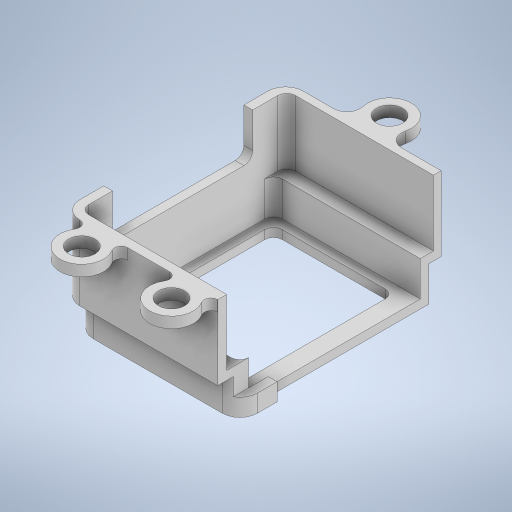
# Autodesk Inventor part: CO-1-06-motorControllersMount
Saved by Autodesk Inventor 2023 (Build 270158000, 158)
## iProperties
Created: 2023-01-24
Part Number: CO-1-06-motorControllersMount
Material: Generic
Document SubType Name: Modeling
Designer: t205b
Density: 1 g/cm^3
Appearance: Default
Author: t205b
Autodesk Inventor part; units mm, degrees
ref_plane "YZ Plane" through (0, 0, 0) normal (1, 0, 0) x (0, 1, 0)
ref_plane "XZ Plane" through (0, 0, 0) normal (0, 1, 0) x (-1, 0, 0)
sketch "Sketch1" plane through (0, 0, 0) normal (0, 1, 0) x (-1, 0, 0)
  arc A0 (31.569, 13.7227) -> (30.069, 12.2227) centre (31.569, 12.2227) ccw
  line L0 (31.569, 13.7227) -> (34.069, 13.7227)
  line L1 (34.069, 13.7227) -> (34.069, 18.9227)
  line L2 (32.069, 20.9227) -> (2.569, 20.9227)
  line L3 (34.069, -13.2773) -> (31.569, -13.2773)
  arc A1 (30.069, -11.7773) -> (31.569, -13.2773) centre (31.569, -11.7773) ccw
  arc A2 (34.069, 18.9227) -> (32.069, 20.9227) centre (32.069, 18.9227) ccw
  arc A3 (34.0195, 22.4149) -> (32.069, 23.9727) centre (32.069, 21.9727) ccw
  line L4 (32.069, 23.9727) -> (-23.931, 23.9727)
  arc A4 (-23.931, 23.9727) -> (-25.931, 21.9727) centre (-23.931, 21.9727) ccw
  line L5 (-25.931, 21.9727) -> (-25.931, -21.0273)
  arc A5 (-25.931, -21.0273) -> (-23.931, -23.0273) centre (-23.931, -21.0273) ccw
  line L6 (-23.931, -23.0273) -> (32.069, -23.0273)
  arc A6 (32.069, -23.0273) -> (33.899, -21.8341) centre (32.069, -21.0273) ccw
  arc A7 (32.069, -20.2773) -> (34.069, -18.2773) centre (32.069, -18.2773) ccw
  line L7 (32.069, -20.2773) -> (0.569, -20.2773)
  line L8 (34.069, -13.2773) -> (34.069, 13.7227)
  line L9 (0.569, -22.2773) -> (0.569, 18.9227)
  line L10 (30.069, -11.7773) -> (30.069, 12.2227)
  line L11 (34.069, -18.2773) -> (34.069, -13.2773)
  line L12 (2.569, 22.9227) -> (32.069, 22.9227)
  line L13 (0.569, -22.2773) -> (32.069, -22.2773)
  arc A8 (32.069, -22.2773) -> (36.069, -18.2773) centre (32.069, -18.2773) ccw
  line L14 (36.069, -18.2773) -> (36.069, 18.9227)
  arc A9 (2.569, 20.9227) -> (0.569, 18.9227) centre (2.569, 18.9227) ccw
  line L15 (-1.431, 14.4227) -> (-1.431, 18.9227)
  arc A10 (2.569, 22.9227) -> (-1.431, 18.9227) centre (2.569, 18.9227) ccw
  arc A11 (36.069, 18.9227) -> (32.069, 22.9227) centre (32.069, 18.9227) ccw
  line L16 (-1.431, 14.4227) -> (0.569, 14.4227)
  point P0 (0.569, 20.9227)
  dimension "d8" = 2
  dimension "d9" = 2
  dimension "d66" = 2
  dimension "d67" = 2
  dimension "d68" = 4.5
  dimension "d69" = 4
  constraints: 35 end point, 27 point on circle, 12 centre point, 8 vertical, 6 horizontal, 4 point on line, 3 tangent, 2 perpendicular, 1 collinear, 9 other
  measures "d8" distance between parallel lines of L2 L12
  measures "d9" distance between parallel lines of L7 L13
  measures "d66" radius of A9
  measures "d67" radial gap between concentric circles of A9 A10
  measures "d68" distance of L15.start L15.end
  measures "d69" radius of A11
extrude "Extrusion3" add sketch "Sketch1" against normal blind 2 contours L0 L8 L3 A1 L10 A0 | A0 L10 A1 L3 L11 A7 L7 L9 A9 L2 A2 L1 L0 | L1 A2 L2 A9 L9 L16 L15 A10 L12 A11 L14 A8 L13 L7 A7 L11 L8
ref_plane "Work Plane1" through (0, 8, 0) normal (0, 1, 0) x (1, 0, 0)
extrude "Extrusion4" add sketch "Sketch1" along normal blind 8 contours L1 A2 L2 A9 L9 L16 L15 A10 L12 A11 L14 A8 L13 L7 A7 L11 L8
sketch "Sketch2" plane through (0, 8, 0) normal (0, 1, 0) x (1, 0, 0)
  line L0 (-0.569, 22.2773) -> (-0.569, 22.2773) projected
  line L1 (-0.569, 22.2773) -> (-0.569, 22.2773)
  line L2 (-36.069, -21.9727) -> (-36.069, 21.0273)
  line L3 (-32.069, -25.9727) -> (-0.569, -25.9727)
  line L4 (-0.569, -14.4227) -> (-0.569, -18.9227) projected
  line L5 (-0.569, -25.9727) -> (-0.569, -18.9227)
  line L6 (-0.569, -14.4227) -> (-0.569, 20.2773) projected
  line L7 (-0.569, 25.0273) -> (-32.069, 25.0273)
  line L8 (-0.569, 23.2773) -> (-32.069, 23.2773)
  line L9 (-32.069, 22.2773) -> (-0.569, 22.2773) projected
  arc A0 (-36.069, -21.9727) -> (-32.069, -25.9727) centre (-32.069, -21.9727) ccw
  line L10 (-0.569, -23.9227) -> (-32.069, -23.9227)
  line L11 (-34.069, -21.9227) -> (-34.069, 21.2773)
  line L12 (-34.069, 18.2773) -> (-34.069, -18.9227) projected
  arc A1 (-32.069, 23.2773) -> (-34.069, 21.2773) centre (-32.069, 21.2773) ccw
  arc A2 (-32.069, 25.0273) -> (-36.069, 21.0273) centre (-32.069, 21.0273) ccw
  arc A3 (-34.069, -21.9227) -> (-32.069, -23.9227) centre (-32.069, -21.9227) ccw
  line L13 (-34.069, -18.9227) -> (-34.069, 18.2773) projected
  line L14 (-36.069, 18.2773) -> (-36.069, -18.9227) projected
  line L15 (-32.069, 20.2773) -> (-0.569, 20.2773) projected
  line L16 (-2.569, -20.9227) -> (-32.069, -20.9227) projected
  line L17 (-32.069, -22.9227) -> (-2.569, -22.9227) projected
  line L18 (-0.569, 25.0273) -> (-0.569, 22.2773)
  line L19 (-0.569, 20.2773) -> (-0.569, 22.2773) projected
  line L20 (-0.569, 20.2773) -> (-32.069, 20.2773) projected
  arc A4 (-32.069, 20.2773) -> (-34.069, 18.2773) centre (-32.069, 18.2773) ccw projected
  line L21 (-34.069, 18.2773) -> (-34.069, -18.9227) projected
  arc A5 (-34.069, -18.9227) -> (-32.069, -20.9227) centre (-32.069, -18.9227) ccw projected
  line L22 (-32.069, -20.9227) -> (-2.569, -20.9227) projected
  arc A6 (-2.569, -20.9227) -> (-0.569, -18.9227) centre (-2.569, -18.9227) ccw projected
  line L23 (-0.569, -18.9227) -> (-0.569, -14.4227) projected
  line L24 (-0.569, -14.4227) -> (-0.569, 20.2773) projected
  dimension "d79" = 43
  dimension "d80" = 31.5
  dimension "d81" = 4
  dimension "d83" = 4.75
  dimension "d85" = 1
  dimension "d87" = 1
  constraints: 18 end point, 8 point on circle, 6 tangent, 4 centre point, 4 collinear, 3 parallel, 3 point on line, 2 equal radius, 2 perpendicular, 2 vertical, 1 horizontal, 1 other
  measures "d79" distance of L2.start L2.end
  measures "d80" distance of L10.start L10.end
  measures "d81" radius of A0
  measures "d83" distance between parallel lines of L15 L7
  measures "d85" distance between parallel lines of L10 L17
  measures "d87" distance between parallel lines of L9 L8
extrude "Extrusion7" add sketch "Sketch2" against normal blind 2 contours L2 A2 L7 L18 L8 A1 L11 A3 L10 L5 L3 A0 | L10 A3 L11 A5 L16 A6 L5 | L18 L19 L15 A4 L11 A1 L8
extrude "Extrusion8" add sketch "Sketch2" along normal blind 15 contours L2 A2 L7 L18 L8 A1 L11 A3 L10 L5 L3 A0
sketch "Sketch5" plane through (0, 23, 0) normal (0, 1, 0) x (1, 0, 0)
  circle A0 centre (-17.319, 30.0273) radius 5
  circle A1 centre (-17.319, 30.0273) radius 3
  arc A2 (-12.4777, 28.7773) -> (-9.573, 25.0273) centre (-9.573, 28.0273) ccw
  arc A3 (-25.0649, 25.0273) -> (-22.1602, 28.7773) centre (-25.0649, 28.0273) ccw
  circle A4 centre (-6.0917, -30.9727) radius 5
  circle A5 centre (-6.0917, -30.9727) radius 3
  arc A6 (-10.305, -28.2804) -> (-11.569, -25.9727) centre (-11.569, -27.4727) ccw
  arc A7 (-0.6145, -25.9727) -> (-1.8785, -28.2804) centre (-0.6145, -27.4727) ccw
  circle A8 centre (-26.5917, -30.9727) radius 5
  circle A9 centre (-26.5917, -30.9727) radius 3
  arc A10 (-21.1145, -25.9727) -> (-22.3785, -28.2804) centre (-21.1145, -27.4727) ccw
  line L0 (-11.569, -25.9727) -> (-0.6145, -25.9727)
  arc A11 (-30.805, -28.2804) -> (-32.069, -25.9727) centre (-32.069, -27.4727) ccw
  line L1 (-32.069, -25.9727) -> (-0.569, -25.9727) projected
  arc A12 (-36.069, -21.9727) -> (-32.069, -25.9727) centre (-32.069, -21.9727) ccw projected
  line L2 (-0.569, -22.3868) -> (-0.569, -25.9727) projected
  line L3 (-32.069, -25.9727) -> (-0.569, -25.9727)
  line L4 (-0.569, 25.0273) -> (-32.069, 25.0273) projected
  line L5 (-36.069, 21.0273) -> (-36.069, -21.9727) projected
  point P0 (0, 0)
  point P1 (-6.0917, -25.9727)
  point P2 (-26.5917, -25.9727)
  dimension "d34" = 10
  dimension "d35" = 6
  dimension "d38" = 3
  dimension "d39" = 3
  dimension "d40" = 10
  dimension "d41" = 6
  dimension "d42" = 3
  dimension "d43" = 3
  dimension "d44" = 10
  dimension "d45" = 6
  dimension "d47" = 3
  dimension "d49" = 20.5
  dimension "d88" = 3
  dimension "d89" = 18.75
  constraints: 18 point on circle, 15 tangent, 12 centre point, 5 end point, 3 coincident, 3 point on line, 1 collinear, 1 horizontal
  measures "d34" diameter of A0
  measures "d35" diameter of A1
  measures "d38" radius of A3
  measures "d39" radius of A2
  measures "d40" diameter of A4
  measures "d41" diameter of A5
  measures "d42" diameter of A6
  measures "d43" diameter of A7
  measures "d44" diameter of A8
  measures "d45" diameter of A9
  measures "d47" diameter of A10
  measures "d49" distance of A4.centre A8.centre
  measures "d88" diameter of A11
  measures "d89" distance from line of L5 A0.centre
extrude "Extrusion10" add sketch "Sketch5" against normal blind 2.5
sketch "Sketch6" plane through (0, -2, 0) normal (0, -1, 0) x (1, 0, 0)
  line L0 (-0.569, -22.2773) -> (-0.569, 14.4227) projected
  line L1 (-2.569, 22.9227) -> (-32.069, 22.9227) projected
  arc A0 (-32.069, 22.9227) -> (-36.069, 18.9227) centre (-32.069, 18.9227) ccw projected
  line L2 (-36.069, 18.9227) -> (-36.069, -18.2773) projected
  arc A1 (-36.069, -18.2773) -> (-32.069, -22.2773) centre (-32.069, -18.2773) ccw projected
  line L3 (-32.069, -22.2773) -> (-0.569, -22.2773) projected
  line L4 (-30.069, 18.9227) -> (-6.569, 18.9227)
  line L5 (-4.569, 16.9227) -> (-4.569, -16.2773)
  line L6 (-6.569, -18.2773) -> (-30.069, -18.2773)
  line L7 (-32.069, -16.2773) -> (-32.069, 16.9227)
  arc A2 (-6.569, -18.2773) -> (-4.569, -16.2773) centre (-6.569, -16.2773) ccw
  arc A3 (-32.069, -16.2773) -> (-30.069, -18.2773) centre (-30.069, -16.2773) ccw
  arc A4 (-30.069, 18.9227) -> (-32.069, 16.9227) centre (-30.069, 16.9227) ccw
  arc A5 (-4.569, 16.9227) -> (-6.569, 18.9227) centre (-6.569, 16.9227) ccw
  line L8 (-0.569, 14.4227) -> (1.431, 14.4227) projected
  line L9 (1.431, 14.4227) -> (1.431, 18.9227) projected
  arc A6 (1.431, 18.9227) -> (-2.569, 22.9227) centre (-2.569, 18.9227) ccw projected
  point P0 (0, 0)
  point P1 (-4.569, 18.9227)
  point P2 (-4.569, -18.2773)
  dimension "d52" = 4
  dimension "d53" = 37.2
  dimension "d54" = 27.5
  dimension "d55" = 4
  dimension "d56" = 2
  constraints: 8 end point, 8 point on circle, 8 tangent, 4 centre point, 4 point on line, 3 equal radius, 3 perpendicular
  measures "d52" distance between parallel lines of L1 L4
  measures "d53" distance of point (-4.569, 18.923) point (-4.569, -18.277)
  measures "d54" distance between parallel lines of L5 L7
  measures "d55" distance between parallel lines of L0 L5
  measures "d56" radius of A2
extrude "Extrusion11" cut sketch "Sketch6" against normal blind 2 contours L4 A5 L5 A2 L6 A3 L7 A4
sketch "Sketch7" plane through (-36.069, -2, -18.2773) normal (-1, 0, 0) x (0, 0, 1)
  line L0 (2.75, 25) -> (34.75, 25)
  line L1 (34.75, 25) -> (34.75, 17)
  line L2 (32.75, 15) -> (4.75, 15)
  line L3 (2.75, 17) -> (2.75, 25)
  arc A0 (2.75, 17) -> (4.75, 15) centre (4.75, 17) ccw
  arc A1 (32.75, 15) -> (34.75, 17) centre (32.75, 17) ccw
  line L4 (40.25, 8) -> (40.25, 25) projected
  line L5 (-2.75, 25) -> (40.25, 25) projected
  point P0 (18.2773, 2)
  point P1 (34.75, 21)
  dimension "d59" = 2
  dimension "d61" = 32
  dimension "d90" = 5.5
  dimension "d91" = 10
  constraints: 8 end point, 4 point on circle, 4 tangent, 2 centre point, 2 parallel, 1 collinear, 1 equal radius, 1 horizontal, 1 midpoint, 1 perpendicular
  measures "d59" radius of A0
  measures "d61" distance from line of point (34.75, 21) L3
  measures "d90" distance between parallel lines of L4 L1
  measures "d91" distance between parallel lines of L0 L2
extrude "Extrusion12" cut sketch "Sketch7" against normal blind 6
sketch "Sketch8" plane through (0, 8, 0) normal (0, 1, 0) x (1, 0, 0)
  line L0 (-0.569, -14.4227) -> (-0.569, -18.9227) projected
  line L1 (1.431, -14.4227) -> (-0.569, -14.4227) projected
  line L2 (1.431, -18.9227) -> (1.431, -14.4227) projected
  arc A0 (-0.569, -22.3868) -> (1.431, -18.9227) centre (-2.569, -18.9227) ccw projected
  line L3 (-0.569, -23.9727) -> (-0.569, -18.9227) projected
  point P0 (0, 0)
  point P1 (-0.4025, -22.2852)
  point P2 (-0.4025, -22.2852)
  point P3 (-2.569, -22.9227)
  point P4 (-0.569, -22.3868)
extrude "Extrusion13" cut sketch "Sketch8" against normal blind 6
equation "\"shrink\" = 0.25"
body "Solid2"
